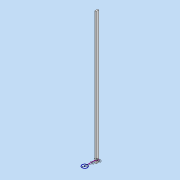
# Autodesk Inventor part: spiral block
Saved by Autodesk Inventor 2020 (Build 240168000, 168)
## iProperties
Created: 2020-12-17
Part Number: spiral block
Material: Generic
Document SubType Name: Modeling
Designer: solar
Density: 1 g/cm^3
Appearance: Default
Author: solar
Autodesk Inventor part; units mm, degrees
ref_plane "YZ Plane" through (0, 0, 0) normal (1, 0, 0) x (0, 1, 0)
ref_plane "XZ Plane" through (0, 0, 0) normal (0, 1, 0) x (-1, 0, 0)
ref_plane "XY Plane" through (0, 0, 0) normal (0, 0, 1) x (1, 0, 0)
sketch "Sketch1" plane through (0, 0, 0) normal (0, 1, 0) x (-1, 0, 0)
  circle A0 centre (0, 0) radius 10
  line L0 (0, -10) -> (0, -40)
  line L1 (0, -40) -> (0, -50)
  line L2 (0, -40) -> (-5, -40)
  line L3 (-5, -40) -> (-5, -50)
  line L4 (-5, -50) -> (0, -50)
  dimension "d0" = 20
  dimension "d1" = 30
  dimension "d2" = 10
  dimension "d3" = 5
  dimension "d4" = 10
  constraints: 10 end point, 3 vertical, 1 coincident, 1 perpendicular, 1 vertical alignment, 2 other
  measures "d1" distance of L0.start L0.end
  measures "d2" distance of L0.end L1.end
  measures "d3" distance of L0.end L2.end
  measures "d4" distance of L2.end L3.end
extrude "Extrusion1" add sketch "Sketch1" along normal blind 500 contours L1 L4 L3 L2
extrude "Extrusion2" add sketch "Sketch1" against normal blind 10 contours L1 L4 L3 L2
body "Solid1"
